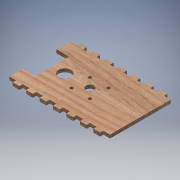
# Autodesk Inventor part: ArmMount
Saved by Autodesk Inventor 2019 (Build 230136000, 136)
## iProperties
Created: 2019-01-16
Part Number: ArmMount
Material: Wood (Birch)
Document SubType Name: Modeling
Designer: nxgam
Density: 0.55 g/cm^3
Appearance: Birch - Natural Polished
Author: nxgam
Autodesk Inventor part; units mm, degrees
ref_plane "YZ Plane" through (0, 0, 0) normal (1, 0, 0) x (0, 1, 0)
ref_plane "XZ Plane" through (0, 0, 0) normal (0, 1, 0) x (-1, 0, 0)
ref_plane "XY Plane" through (0, 0, 0) normal (0, 0, 1) x (1, 0, 0)
sketch "Sketch1" plane through (0, 0, 0) normal (0, 1, 0) x (-1, 0, 0)
  line L0 (-76.2, 50.8) -> (76.2, 50.8)
  line L1 (76.2, 50.8) -> (76.2, -50.8)
  line L2 (76.2, -50.8) -> (-76.2, -50.8)
  line L3 (-76.2, -50.8) -> (-76.2, 50.8)
  line L4 (-76.2, 50.8) -> (76.2, -50.8) construction
  line L5 (76.2, 50.8) -> (-76.2, -50.8) construction
  point P0 (0, 0)
  dimension "d0" = 152.4
  dimension "d1" = 101.6
  constraints: 12 end point, 2 midpoint, 2 parallel, 1 horizontal, 1 perpendicular
  measures "d0" distance of L1.end L2.end
  measures "d1" distance of L0.end L1.end
extrude "Extrusion1" add sketch "Sketch1" along normal blind 5.08
sketch "Sketch2" plane through (0, 5.08, 0) normal (0, 1, 0) x (1, 0, 0)
  line L0 (-76.2, -50.8) -> (76.2, -50.8) projected
  line L1 (76.2, -50.8) -> (76.2, 50.8) projected
  line L2 (76.2, 50.8) -> (-76.2, 50.8) projected
  line L3 (-76.2, 50.8) -> (-76.2, -50.8) projected
  line L4 (-76.2, -50.8) -> (-66.04, -50.8)
  line L5 (-66.04, -50.8) -> (-66.04, -45.72)
  line L6 (-66.04, -45.72) -> (-76.2, -45.72)
  line L7 (-76.2, -45.72) -> (-76.2, -50.8)
  line L8 (-55.88, -50.8) -> (-45.72, -50.8)
  line L9 (-45.72, -50.8) -> (-45.72, -45.72)
  line L10 (-45.72, -45.72) -> (-55.88, -45.72)
  line L11 (-55.88, -45.72) -> (-55.88, -50.8)
  line L12 (-35.56, -50.8) -> (-25.4, -50.8)
  line L13 (-25.4, -50.8) -> (-25.4, -45.72)
  line L14 (-25.4, -45.72) -> (-35.56, -45.72)
  line L15 (-35.56, -45.72) -> (-35.56, -50.8)
  line L16 (-15.24, -50.8) -> (-5.08, -50.8)
  line L17 (-5.08, -50.8) -> (-5.08, -45.72)
  line L18 (-5.08, -45.72) -> (-15.24, -45.72)
  line L19 (-15.24, -45.72) -> (-15.24, -50.8)
  line L20 (5.08, -50.8) -> (15.24, -50.8)
  line L21 (15.24, -50.8) -> (15.24, -45.72)
  line L22 (15.24, -45.72) -> (5.08, -45.72)
  line L23 (5.08, -45.72) -> (5.08, -50.8)
  line L24 (25.4, -50.8) -> (35.56, -50.8)
  line L25 (35.56, -50.8) -> (35.56, -45.72)
  line L26 (35.56, -45.72) -> (25.4, -45.72)
  line L27 (25.4, -45.72) -> (25.4, -50.8)
  line L28 (45.72, -50.8) -> (55.88, -50.8)
  line L29 (55.88, -50.8) -> (55.88, -45.72)
  line L30 (55.88, -45.72) -> (45.72, -45.72)
  line L31 (45.72, -45.72) -> (45.72, -50.8)
  line L32 (66.04, -50.8) -> (76.2, -50.8)
  line L33 (76.2, -50.8) -> (76.2, -45.72)
  line L34 (76.2, -45.72) -> (66.04, -45.72)
  line L35 (66.04, -45.72) -> (66.04, -50.8)
  line L36 (-76.2, 50.8) -> (-76.2, -50.8) construction
  line L37 (-76.2, 0) -> (76.2, 0) construction
  line L38 (-76.2, 50.8) -> (76.2, 50.8)
  line L39 (-76.2, 50.8) -> (-66.04, 50.8)
  line L40 (-66.04, 50.8) -> (-66.04, 45.72)
  line L41 (-66.04, 45.72) -> (-76.2, 45.72)
  line L42 (-76.2, 45.72) -> (-76.2, 50.8)
  line L43 (-55.88, 50.8) -> (-45.72, 50.8)
  line L44 (-45.72, 50.8) -> (-45.72, 45.72)
  line L45 (-45.72, 45.72) -> (-55.88, 45.72)
  line L46 (-55.88, 45.72) -> (-55.88, 50.8)
  line L47 (-35.56, 50.8) -> (-25.4, 50.8)
  line L48 (-25.4, 50.8) -> (-25.4, 45.72)
  line L49 (-25.4, 45.72) -> (-35.56, 45.72)
  line L50 (-35.56, 45.72) -> (-35.56, 50.8)
  line L51 (-15.24, 50.8) -> (-5.08, 50.8)
  line L52 (-5.08, 50.8) -> (-5.08, 45.72)
  line L53 (-5.08, 45.72) -> (-15.24, 45.72)
  line L54 (-15.24, 45.72) -> (-15.24, 50.8)
  line L55 (5.08, 50.8) -> (15.24, 50.8)
  line L56 (15.24, 50.8) -> (15.24, 45.72)
  line L57 (15.24, 45.72) -> (5.08, 45.72)
  line L58 (5.08, 45.72) -> (5.08, 50.8)
  line L59 (25.4, 50.8) -> (35.56, 50.8)
  line L60 (35.56, 50.8) -> (35.56, 45.72)
  line L61 (35.56, 45.72) -> (25.4, 45.72)
  line L62 (25.4, 45.72) -> (25.4, 50.8)
  line L63 (45.72, 50.8) -> (55.88, 50.8)
  line L64 (55.88, 50.8) -> (55.88, 45.72)
  line L65 (55.88, 45.72) -> (45.72, 45.72)
  line L66 (45.72, 45.72) -> (45.72, 50.8)
  line L67 (66.04, 50.8) -> (76.2, 50.8)
  line L68 (76.2, 50.8) -> (76.2, 45.72)
  line L69 (76.2, 45.72) -> (66.04, 45.72)
  line L70 (66.04, 45.72) -> (66.04, 50.8)
  point P0 (0, 0)
  point P1 (0, 0)
  dimension "d11" = 10.16
  dimension "d12" = 5.08
  dimension "d13" = 0
  dimension "d16" = 20.32
  constraints: 132 end point, 41 symmetric about line, 2 horizontal, 2 midpoint, 2 parallel, 2 point on line, 1 coincident, 1 perpendicular, 63 other
  measures "d11" distance of L5.end L6.end
  measures "d12" distance of L6.end L4.start
  measures "d13" distance between parallel lines of L3 L7
  measures "d16" distance of L0.start point (-55.88, -50.8)
hole "Hole1" at (0, 5.08, 0) direction (0, -1, 0) diameter 12.5 end through all
extrude "Extrusion2" cut sketch "Sketch2" against normal blind 5.08 contours L5 L6 L3 L41 L40 L2 L46 L45 L44 L50 L49 L48 L54 L53 L52 L58 L57 L56 L62 L61 L60 L66 L65 L64 L70 L69 L1 L34 L35 L0 L29 L30 L31 L25 L26 L27 L21 L22 L23 L17 L18 L19 L13 L14 L15 L9 L10 L11 keep common part
sketch "Sketch3" plane through (0, 0, 0) normal (0, -1, 0) x (1, 0, 0)
  circle A0 centre (-38.1, 0) radius 9.525
  line L0 (0, 0) -> (-38.1, 0) construction
  dimension "d23" = 19.05
  dimension "d24" = 38.1
  constraints: 2 end point, 1 centre point, 1 horizontal
  measures "d23" diameter of A0
  measures "d24" distance of L0.start L0.end
extrude "Extrusion3" cut sketch "Sketch3" against normal blind 25.4
sketch "Sketch4" plane through (0, 0, 0) normal (0, -1, 0) x (1, 0, 0)
  circle A0 centre (13.97, -13.97) radius 2.5
  circle A1 centre (-13.97, -13.97) radius 2.5
  circle A2 centre (-13.97, 13.97) radius 2.5
  circle A3 centre (13.97, 13.97) radius 2.5
  point P0 (0, 0)
  constraints: 4 centre point, 8 other
extrude "Extrusion4" cut sketch "Sketch4" against normal blind 25.4
sketch "Sketch5" plane through (0, 0, 0) normal (0, -1, 0) x (1, 0, 0)
  circle A0 centre (-13.97, 13.97) radius 2.5 projected
  circle A1 centre (13.97, -13.97) radius 2.5 projected
  circle A2 centre (-13.97, -13.97) radius 2.5 projected
  circle A3 centre (13.97, 13.97) radius 2.5 projected
  circle A4 centre (-38.1, 0) radius 9.525 projected
  circle A5 centre (0, 0) radius 6.25 projected
  line L0 (66.04, -45.72) -> (66.04, -50.8) construction
  line L1 (76.2, -45.72) -> (66.04, -45.72) construction
  line L2 (76.2, -45.72) -> (76.2, 45.72) construction
  line L3 (66.04, 45.72) -> (76.2, 45.72) construction
  line L4 (66.04, 50.8) -> (66.04, 45.72) construction
  line L5 (66.04, 50.8) -> (55.88, 50.8) construction
  line L6 (55.88, 45.72) -> (55.88, 50.8) construction
  line L7 (45.72, 45.72) -> (55.88, 45.72) construction
  line L8 (45.72, 50.8) -> (45.72, 45.72) construction
  line L9 (45.72, 50.8) -> (35.56, 50.8) construction
  line L10 (35.56, 45.72) -> (35.56, 50.8) projected
  line L11 (25.4, 45.72) -> (35.56, 45.72) projected
  line L12 (25.4, 50.8) -> (25.4, 45.72) projected
  line L13 (25.4, 50.8) -> (15.24, 50.8) projected
  line L14 (15.24, 45.72) -> (15.24, 50.8) projected
  line L15 (5.08, 45.72) -> (15.24, 45.72) projected
  line L16 (5.08, 50.8) -> (5.08, 45.72) projected
  line L17 (5.08, 50.8) -> (-5.08, 50.8) projected
  line L18 (-5.08, 45.72) -> (-5.08, 50.8) projected
  line L19 (-15.24, 45.72) -> (-5.08, 45.72) projected
  line L20 (-15.24, 50.8) -> (-15.24, 45.72) projected
  line L21 (-15.24, 50.8) -> (-25.4, 50.8) projected
  line L22 (-25.4, 45.72) -> (-25.4, 50.8) projected
  line L23 (-35.56, 45.72) -> (-25.4, 45.72) projected
  line L24 (-35.56, 50.8) -> (-35.56, 45.72) projected
  line L25 (-35.56, 50.8) -> (-45.72, 50.8) projected
  line L26 (-45.72, 45.72) -> (-45.72, 50.8) projected
  line L27 (-55.88, 45.72) -> (-45.72, 45.72) projected
  line L28 (-55.88, 50.8) -> (-55.88, 45.72) projected
  line L29 (-55.88, 50.8) -> (-66.04, 50.8) projected
  line L30 (-66.04, 45.72) -> (-66.04, 50.8) projected
  line L31 (-76.2, 45.72) -> (-66.04, 45.72) projected
  line L32 (-76.2, 45.72) -> (-76.2, -45.72) projected
  line L33 (-66.04, -45.72) -> (-76.2, -45.72) projected
  line L34 (-66.04, -50.8) -> (-66.04, -45.72) projected
  line L35 (-66.04, -50.8) -> (-55.88, -50.8) projected
  line L36 (-55.88, -45.72) -> (-55.88, -50.8) projected
  line L37 (-45.72, -45.72) -> (-55.88, -45.72) projected
  line L38 (-45.72, -50.8) -> (-45.72, -45.72) projected
  line L39 (-45.72, -50.8) -> (-35.56, -50.8) projected
  line L40 (-35.56, -45.72) -> (-35.56, -50.8) projected
  line L41 (-25.4, -45.72) -> (-35.56, -45.72) projected
  line L42 (-25.4, -50.8) -> (-25.4, -45.72) projected
  line L43 (-25.4, -50.8) -> (-15.24, -50.8) projected
  line L44 (-15.24, -45.72) -> (-15.24, -50.8) projected
  line L45 (-5.08, -45.72) -> (-15.24, -45.72) projected
  line L46 (-5.08, -50.8) -> (-5.08, -45.72) projected
  line L47 (-5.08, -50.8) -> (5.08, -50.8) projected
  line L48 (5.08, -45.72) -> (5.08, -50.8) projected
  line L49 (15.24, -45.72) -> (5.08, -45.72) projected
  line L50 (15.24, -50.8) -> (15.24, -45.72) projected
  line L51 (15.24, -50.8) -> (25.4, -50.8) projected
  line L52 (25.4, -45.72) -> (25.4, -50.8) projected
  line L53 (35.56, -45.72) -> (25.4, -45.72) projected
  line L54 (35.56, -50.8) -> (35.56, -45.72) projected
  line L55 (35.56, -50.8) -> (45.72, -50.8) construction
  line L56 (45.72, -45.72) -> (45.72, -50.8) construction
  line L57 (55.88, -45.72) -> (45.72, -45.72) construction
  line L58 (55.88, -50.8) -> (55.88, -45.72) construction
  line L59 (55.88, -50.8) -> (66.04, -50.8) construction
  line L60 (-76.2, -45.72) -> (-76.2, 45.72) projected
  line L61 (-76.2, 25.4) -> (-57.15, 25.4)
  line L62 (-57.15, 25.4) -> (-57.15, -25.4)
  line L63 (-57.15, -25.4) -> (-76.2, -25.4)
  line L64 (-76.2, -25.4) -> (-76.2, 25.4)
  line L65 (-57.15, 0) -> (-76.2, 0) construction
  line L66 (-76.2, 25.4) -> (-57.15, 25.4)
  line L67 (-57.15, 25.4) -> (-57.15, -25.4)
  line L68 (-57.15, -25.4) -> (-76.2, -25.4)
  line L69 (-76.2, -25.4) -> (-76.2, 25.4)
  dimension "d29" = 50.8
  dimension "d30" = 19.05
  constraints: 18 end point, 4 parallel, 3 midpoint, 2 horizontal, 2 perpendicular, 1 point on line
  measures "d29" distance of L61.end L62.end
  measures "d30" distance between parallel lines of L64 L62
extrude "Extrusion5" cut sketch "Sketch5" against normal blind 25.4 contours L61 L62 L63 L32
fillet "Fillet1" radius 6.35 4 edges at (-57.15, 2.54, -25.4) (-76.2, 2.54, -25.4) (-57.15, 2.54, 25.4) (-76.2, 2.54, 25.4)
equation "\"d16\" = 2 * d11"
body "Solid1"
